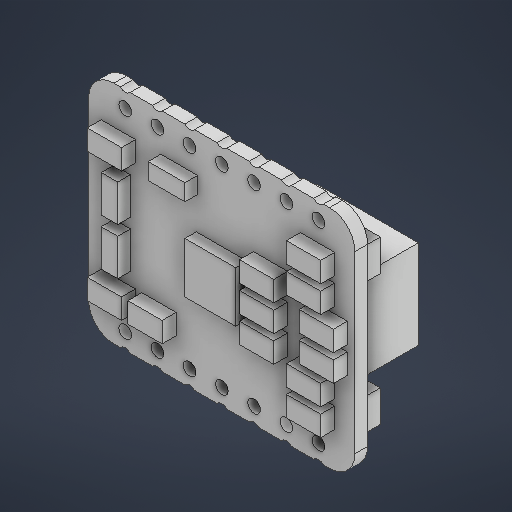
# Autodesk Inventor part: PCB
Saved by Autodesk Inventor 2027 (Build 310192000, 192)
## iProperties
Created: 2026-07-04
Part Number: PCB
Material: Genérico
Document SubType Name: Modeling
Designer: marcu
Density: 1 g/cm^3
Appearance: Padrão
Author: marcu
Autodesk Inventor part; units mm, degrees
ref_plane "YZ Plane" through (0, 0, 0) normal (1, 0, 0) x (0, 1, 0)
ref_plane "XZ Plane" through (0, 0, 0) normal (0, 1, 0) x (-1, 0, 0)
ref_plane "XY Plane" through (0, 0, 0) normal (0, 0, 1) x (1, 0, 0)
sketch "Esboço1" plane through (0, 0, 0) normal (0, 0, 1) x (1, 0, 0)
  line L0 (-10.5, 8.9) -> (10.5, 8.9)
  line L1 (10.5, 8.9) -> (10.5, -8.9)
  line L2 (10.5, -8.9) -> (-10.5, -8.9)
  line L3 (-10.5, -8.9) -> (-10.5, 8.9)
  line L4 (-10.5, 8.9) -> (10.5, -8.9) construction
  line L5 (10.5, 8.9) -> (-10.5, -8.9) construction
  point P0 (0, 0)
  dimension "d0" = 21
  dimension "d1" = 17.8
  constraints: 12 end point, 2 midpoint, 2 parallel, 1 horizontal, 1 perpendicular
  measures "d0" distance of L1.end L2.end
  measures "d1" distance of L0.end L1.end
extrude "Extrusão1" add sketch "Esboço1" along normal blind 1
fillet "Arredondamento1" radius 2 4 edges at (10.5, 8.9, 0.5) (10.5, -8.9, 0.5) (-10.5, -8.9, 0.5) (-10.5, 8.9, 0.5)
sketch "Esboço2" plane through (0, 0, 1) normal (0, 0, 1) x (1, 0, 0)
  line L0 (10.5, 8.9) -> (-10.5, 8.9) construction
  line L1 (-10.5, 8.9) -> (-10.5, -8.9) construction
  line L2 (-10.5, -8.9) -> (10.5, -8.9) construction
  line L3 (10.5, -8.9) -> (10.5, 8.9) construction
  line L4 (10.5, 8.9) -> (-10.5, -8.9) construction
  line L5 (-10.5, 8.9) -> (10.5, -8.9) construction
  circle A0 centre (7.63, -7.62) radius 0.5
  circle A1 centre (5.09, -7.62) radius 0.5
  circle A2 centre (2.55, -7.62) radius 0.5
  circle A3 centre (0.01, -7.62) radius 0.5
  circle A4 centre (-2.53, -7.62) radius 0.5
  circle A5 centre (-5.07, -7.62) radius 0.5
  circle A6 centre (-7.61, -7.62) radius 0.5
  line L6 (0, 0) -> (4.59, 0) construction
  circle A7 centre (7.63, 7.62) radius 0.5
  circle A8 centre (5.09, 7.62) radius 0.5
  circle A9 centre (2.55, 7.62) radius 0.5
  circle A10 centre (0.01, 7.62) radius 0.5
  circle A11 centre (-2.53, 7.62) radius 0.5
  circle A12 centre (-5.07, 7.62) radius 0.5
  circle A13 centre (-7.61, 7.62) radius 0.5
  dimension "d6" = 21
  dimension "d7" = 17.8
  dimension "d8" = 1
  dimension "d9" = 1.28
  dimension "d10" = 2.87
  dimension "d13" = 2.54
  constraints: 14 centre point, 14 end point, 7 symmetric about line, 3 horizontal, 2 midpoint, 2 parallel, 1 perpendicular, 19 other
  measures "d6" distance of L2.end L1.end
  measures "d7" distance of L1.end L0.end
  measures "d8" diameter of A0
  measures "d9" distance from line of L2 A0.centre
  measures "d10" distance from line of A0.centre L3
  measures "d13" distance of A0.centre A1.centre
extrude "Extrusão2" cut sketch "Esboço2" against normal blind 2
sketch "Esboço3" plane through (0, 0, 1) normal (0, 0, 1) x (1, 0, 0)
  circle A0 centre (7.63, -9.22) radius 0.5
  circle A1 centre (7.63, -7.62) radius 0.5 projected
  line L0 (8.6638, -8.12) -> (6.5962, -8.12) construction
  line L1 (8.6792, -8.72) -> (6.5808, -8.72) construction
  line L2 (-8.5, -8.9) -> (8.5, -8.9) projected
  line L3 (10.5, -6.9) -> (10.5, 6.9) projected
  circle A2 centre (5.09, -9.22) radius 0.5
  line L4 (6.1238, -8.12) -> (4.0562, -8.12) construction
  line L5 (6.1392, -8.72) -> (4.0408, -8.72) construction
  circle A3 centre (2.55, -9.22) radius 0.5
  line L6 (3.5838, -8.12) -> (1.5162, -8.12) construction
  line L7 (3.5992, -8.72) -> (1.5008, -8.72) construction
  circle A4 centre (0.01, -9.22) radius 0.5
  line L8 (1.0438, -8.12) -> (-1.0238, -8.12) construction
  line L9 (1.0592, -8.72) -> (-1.0392, -8.72) construction
  circle A5 centre (-2.53, -9.22) radius 0.5
  line L10 (-1.4962, -8.12) -> (-3.5638, -8.12) construction
  line L11 (-1.4808, -8.72) -> (-3.5792, -8.72) construction
  circle A6 centre (-5.07, -9.22) radius 0.5
  line L12 (-4.0362, -8.12) -> (-6.1038, -8.12) construction
  line L13 (-4.0208, -8.72) -> (-6.1192, -8.72) construction
  circle A7 centre (-7.61, -9.22) radius 0.5
  line L14 (-6.5762, -8.12) -> (-8.6438, -8.12) construction
  line L15 (-6.5608, -8.72) -> (-8.6592, -8.72) construction
  line L16 (2.53, 0) -> (-2.53, 0) construction
  circle A8 centre (7.63, 9.22) radius 0.5
  line L17 (8.6792, 8.72) -> (6.5808, 8.72) construction
  line L18 (-8.5, 8.9) -> (8.5, 8.9)
  circle A9 centre (5.09, 9.22) radius 0.5
  line L19 (6.1392, 8.72) -> (4.0408, 8.72) construction
  circle A10 centre (2.55, 9.22) radius 0.5
  line L20 (3.5992, 8.72) -> (1.5008, 8.72) construction
  circle A11 centre (0.01, 9.22) radius 0.5
  line L21 (1.0592, 8.72) -> (-1.0392, 8.72) construction
  circle A12 centre (-2.53, 9.22) radius 0.5
  line L22 (-1.4808, 8.72) -> (-3.5792, 8.72) construction
  circle A13 centre (-5.07, 9.22) radius 0.5
  line L23 (-4.0208, 8.72) -> (-6.1192, 8.72) construction
  circle A14 centre (-7.61, 9.22) radius 0.5
  line L24 (-6.5608, 8.72) -> (-8.6592, 8.72) construction
  point P0 (0, 0)
  point P1 (7.63, -8.12)
  point P2 (7.63, -8.72)
  point P3 (5.09, -8.72)
  point P4 (5.09, -8.12)
  point P5 (5.09, -7.62)
  point P6 (5.96, -8.9)
  point P7 (2.55, -8.72)
  point P8 (2.55, -8.12)
  point P9 (2.55, -7.62)
  point P10 (3.42, -8.9)
  point P11 (0.01, -8.72)
  point P12 (0.01, -8.12)
  point P13 (0.01, -7.62)
  point P14 (0.88, -8.9)
  point P15 (-2.53, -8.72)
  point P16 (-2.53, -8.12)
  point P17 (-2.53, -7.62)
  point P18 (-1.66, -8.9)
  point P19 (-5.07, -8.72)
  point P20 (-5.07, -8.12)
  point P21 (-5.07, -7.62)
  point P22 (-4.2, -8.9)
  point P23 (-7.61, -8.72)
  point P24 (-7.61, -8.12)
  point P25 (-7.61, -7.62)
  point P26 (-6.74, -8.9)
  point P27 (7.63, 8.72)
  point P28 (5.09, 8.72)
  point P29 (5.96, 8.9)
  point P30 (2.55, 8.72)
  point P31 (3.42, 8.9)
  point P32 (0.01, 8.72)
  point P33 (0.88, 8.9)
  point P34 (-2.53, 8.72)
  point P35 (-1.66, 8.9)
  point P36 (-5.07, 8.72)
  point P37 (-4.2, 8.9)
  point P38 (-7.61, 8.72)
  point P39 (-6.74, 8.9)
  dimension "d20" = 1
  dimension "d21" = 0.6
  dimension "d22" = 2.87
  dimension "d25" = 2.54
  constraints: 46 end point, 36 symmetric about line, 18 horizontal, 15 vertical alignment, 3 midpoint, 1 parallel, 95 other
  measures "d21" distance between parallel lines of L0 L1
  measures "d22" distance from line of point (7.63, -9.22) L3
  measures "d25" distance of point (7.63, -9.22) point (5.09, -9.22)
extrude "Extrusão3" cut sketch "Esboço3" against normal blind 2 contours A0 L2 | L2 A0 | A7 L2 | L2 A7 | A6 L2 | L2 A6 | A5 L2 | L2 A5 | A4 L2 | L2 A4 | A3 L2 | L2 A3 | A2 L2 | L2 A2 | A8 L18 | L18 A8 | A14 L18 | L18 A14 | A13 L18 | L18 A13 | A12 L18 | L18 A12 | A11 L18 | L18 A11 | A10 L18 | L18 A10 | A9 L18 | L18 A9
sketch "Esboço4" plane through (0, 0, 1) normal (0, 0, 1) x (1, 0, 0)
  line L0 (2, 2) -> (-2, 2)
  line L1 (-2, 2) -> (-2, -2)
  line L2 (-2, -2) -> (2, -2)
  line L3 (2, -2) -> (2, 2)
  line L4 (2, 2) -> (-2, -2) construction
  line L5 (-2, 2) -> (2, -2) construction
  point P0 (0, 0)
  dimension "d32" = 4
  dimension "d33" = 4
  constraints: 12 end point, 2 midpoint, 2 parallel, 1 horizontal, 1 perpendicular
  measures "d32" distance of L2.end L1.end
  measures "d33" distance of L1.end L0.end
extrude "MPU6050" add sketch "Esboço4" along normal blind 0.9
sketch "Esboço5" plane through (0, 0, 1) normal (0, 0, 1) x (1, 0, 0)
  line L0 (2, 2) -> (2, -2) projected
  line L1 (2.9342, -8.9) -> (4.7058, -8.9) projected
  line L2 (0, 2.9633) -> (0, -2.9633) construction
  line L3 (-2, 2) -> (-2, -2)
  line L4 (5.2, 2.9) -> (2.5, 2.9)
  line L5 (2.5, 2.9) -> (2.5, 1.3)
  line L6 (2.5, 1.3) -> (5.2, 1.3)
  line L7 (5.2, 1.3) -> (5.2, 2.9)
  line L8 (5.2, 2.9) -> (2.5, 1.3) construction
  line L9 (2.5, 2.9) -> (5.2, 1.3) construction
  line L10 (5.2, 0.8) -> (2.5, 0.8)
  line L11 (2.5, 0.8) -> (2.5, -0.8)
  line L12 (2.5, -0.8) -> (5.2, -0.8)
  line L13 (5.2, -0.8) -> (5.2, 0.8)
  line L14 (5.2, 0.8) -> (2.5, -0.8) construction
  line L15 (2.5, 0.8) -> (5.2, -0.8) construction
  line L16 (5.2, -1.3) -> (2.5, -1.3)
  line L17 (2.5, -1.3) -> (2.5, -2.9)
  line L18 (2.5, -2.9) -> (5.2, -2.9)
  line L19 (5.2, -2.9) -> (5.2, -1.3)
  line L20 (5.2, -1.3) -> (2.5, -2.9) construction
  line L21 (2.5, -1.3) -> (5.2, -2.9) construction
  point P0 (0, 0)
  point P1 (3.85, 2.1)
  point P2 (3.85, 0)
  point P3 (3.85, -2.1)
  dimension "d127" = 2.7
  dimension "d128" = 1.6
  dimension "d129" = 0.5
  dimension "d130" = 0.5
  dimension "d131" = 0.5
  dimension "d132" = 6
  constraints: 40 end point, 7 midpoint, 6 parallel, 4 equal length, 3 horizontal, 3 perpendicular, 2 point on line, 2 symmetric about line, 1 vertical
  measures "d127" distance of L6.end L5.end
  measures "d128" distance of L5.end L4.end
  measures "d129" distance between parallel lines of L6 L10
  measures "d130" distance between parallel lines of L12 L16
  measures "d131" distance between parallel lines of L0 L5
  measures "d132" distance between parallel lines of L1 L18
sketch "Esboço7" plane through (0, 0, 0) normal (0, 0, -1) x (-1, 0, 0)
  line L0 (-9, -3.5) -> (-1, -3.5)
  line L1 (-1, -3.5) -> (-1, 3.5)
  line L2 (-1, 3.5) -> (-9, 3.5)
  line L3 (-9, 3.5) -> (-9, -3.5)
  line L4 (-9, -3.5) -> (-1, 3.5) construction
  line L5 (-1, -3.5) -> (-9, 3.5) construction
  line L6 (-10.5, -6.9) -> (-10.5, 6.9) projected
  line L7 (-7.2458, 8.9) -> (-5.4742, 8.9) projected
  point P0 (0, 0)
  point P1 (-5, 0)
  dimension "d48" = 8
  dimension "d49" = 7
  dimension "d50" = 1.5
  dimension "d51" = 5.4
  constraints: 12 end point, 2 midpoint, 2 parallel, 1 horizontal, 1 perpendicular
  measures "d48" distance of L2.end L1.end
  measures "d49" distance of L1.end L0.end
  measures "d50" distance between parallel lines of L3 L6
  measures "d51" distance between parallel lines of L7 L2
extrude "JST" add sketch "Esboço7" along normal blind 5.5
sketch "Esboço8" plane through (0, 0, 0) normal (0, 0, -1) x (-1, 0, 0)
  line L0 (-10, 6.4) -> (-6.5, 6.4)
  line L1 (-6.5, 6.4) -> (-6.5, 3.9)
  line L2 (-6.5, 3.9) -> (-10, 3.9)
  line L3 (-10, 3.9) -> (-10, 6.4)
  line L4 (-10, 6.4) -> (-6.5, 3.9) construction
  line L5 (-6.5, 6.4) -> (-10, 3.9) construction
  line L6 (-10.5, -6.9) -> (-10.5, 6.9) projected
  line L7 (-8.5, 8.9) -> (-8.0142, 8.9) projected
  line L8 (-2, 0) -> (2, 0) construction
  line L9 (2, 2) -> (2, -2) projected
  line L10 (-10, -6.4) -> (-6.5, -6.4)
  line L11 (-6.5, -6.4) -> (-6.5, -3.9)
  line L12 (-6.5, -3.9) -> (-10, -3.9)
  line L13 (-10, -3.9) -> (-10, -6.4)
  line L14 (-10, -6.4) -> (-6.5, -3.9) construction
  line L15 (-6.5, -6.4) -> (-10, -3.9) construction
  line L16 (-8.5, -8.9) -> (-8.0142, -8.9)
  point P0 (0, 0)
  point P1 (-8.25, 5.15)
  point P2 (-8.25, -5.15)
  dimension "d54" = 3.5
  dimension "d55" = 2.5
  dimension "d56" = 0.5
  dimension "d57" = 2.5
  constraints: 28 end point, 7 symmetric about line, 4 midpoint, 2 parallel, 1 horizontal, 1 perpendicular
  measures "d54" distance of L1.end L2.end
  measures "d55" distance of L0.end L1.end
  measures "d56" distance between parallel lines of L6 L3
  measures "d57" distance between parallel lines of L0 L7
extrude "Botões Deslizantes" add sketch "Esboço8" along normal blind 1.5
sketch "Esboço9" plane through (0, 0, 0) normal (0, 0, -1) x (-1, 0, 0)
  line L0 (-0.5, -2.35) -> (1.5, -2.35)
  line L1 (1.5, -2.35) -> (1.5, -0.75)
  line L2 (1.5, -0.75) -> (-0.5, -0.75)
  line L3 (-0.5, -0.75) -> (-0.5, -2.35)
  line L4 (-0.5, -2.35) -> (1.5, -0.75) construction
  line L5 (1.5, -2.35) -> (-0.5, -0.75) construction
  line L6 (-0.5, 0.75) -> (1.5, 0.75)
  line L7 (1.5, 0.75) -> (1.5, 2.35)
  line L8 (1.5, 2.35) -> (-0.5, 2.35)
  line L9 (-0.5, 2.35) -> (-0.5, 0.75)
  line L10 (-0.5, 0.75) -> (1.5, 2.35) construction
  line L11 (1.5, 0.75) -> (-0.5, 2.35) construction
  line L12 (-1, 3.5) -> (-1, -3.5) projected
  line L13 (0.3742, 8.9) -> (2.1458, 8.9) projected
  line L14 (2, -1.7) -> (4, -1.7)
  line L15 (4, -1.7) -> (4, -0.1)
  line L16 (4, -0.1) -> (2, -0.1)
  line L17 (2, -0.1) -> (2, -1.7)
  line L18 (2, -1.7) -> (4, -0.1) construction
  line L19 (4, -1.7) -> (2, -0.1) construction
  line L20 (2, 0.1) -> (4, 0.1)
  line L21 (4, 0.1) -> (4, 1.7)
  line L22 (4, 1.7) -> (2, 1.7)
  line L23 (2, 1.7) -> (2, 0.1)
  line L24 (2, 0.1) -> (4, 1.7) construction
  line L25 (4, 0.1) -> (2, 1.7) construction
  line L26 (5.4542, 8.9) -> (7.2258, 8.9) projected
  point P0 (0, 0)
  point P1 (0.5, -1.55)
  point P2 (0.5, 1.55)
  point P3 (3, -0.9)
  point P4 (3, 0.9)
  dimension "d60" = 2
  dimension "d61" = 1.6
  dimension "d62" = 0.5
  dimension "d63" = 1.5
  dimension "d64" = 6.55
  dimension "d67" = 0.2
  dimension "d68" = 7.2
  dimension "d69" = 0.5
  dimension "d70" = 0.5
  constraints: 48 end point, 8 midpoint, 8 parallel, 6 equal length, 4 horizontal, 4 perpendicular, 1 point on line
  measures "d60" distance of L1.end L2.end
  measures "d61" distance of L0.start L2.end
  measures "d62" distance between parallel lines of L3 L12
  measures "d63" distance between parallel lines of L6 L2
  measures "d64" distance between parallel lines of L13 L8
  measures "d67" distance between parallel lines of L20 L16
  measures "d68" distance between parallel lines of L26 L22
  measures "d69" distance between parallel lines of L23 L7
  measures "d70" distance between parallel lines of L17 L1
extrude "capacitores" add sketch "Esboço9" along normal blind 1.6
sketch "Esboço10" plane through (0, 0, 0) normal (0, 0, -1) x (-1, 0, 0)
  line L0 (-0.8, -6.4) -> (0.8, -6.4)
  line L1 (0.8, -6.4) -> (0.8, -3.7)
  line L2 (0.8, -3.7) -> (-0.8, -3.7)
  line L3 (-0.8, -3.7) -> (-0.8, -6.4)
  line L4 (-0.8, -6.4) -> (0.8, -3.7) construction
  line L5 (0.8, -6.4) -> (-0.8, -3.7) construction
  line L6 (1.3, -6.4) -> (2.6, -6.4)
  line L7 (2.6, -6.4) -> (2.6, -3.5)
  line L8 (2.6, -3.5) -> (1.3, -3.5)
  line L9 (1.3, -3.5) -> (1.3, -6.4)
  line L10 (1.3, -6.4) -> (2.6, -3.5) construction
  line L11 (2.6, -6.4) -> (1.3, -3.5) construction
  line L12 (3.1, -6.4) -> (3.9, -6.4)
  line L13 (3.9, -6.4) -> (3.9, -4.8)
  line L14 (3.9, -4.8) -> (3.1, -4.8)
  line L15 (3.1, -4.8) -> (3.1, -6.4)
  line L16 (3.1, -6.4) -> (3.9, -4.8) construction
  line L17 (3.9, -6.4) -> (3.1, -4.8) construction
  line L18 (-1, 3.5) -> (-1, -3.5) projected
  line L19 (2.1458, -8.9) -> (0.3742, -8.9) projected
  line L20 (4.6858, -8.9) -> (2.9142, -8.9) projected
  line L21 (7.2258, -8.9) -> (5.4542, -8.9) projected
  line L22 (-1.26, 0) -> (1.26, 0) construction
  line L23 (-0.8, 6.4) -> (0.8, 6.4)
  line L24 (0.8, 6.4) -> (0.8, 3.7)
  line L25 (0.8, 3.7) -> (-0.8, 3.7)
  line L26 (-0.8, 3.7) -> (-0.8, 6.4)
  line L27 (-0.8, 6.4) -> (0.8, 3.7) construction
  line L28 (0.8, 6.4) -> (-0.8, 3.7) construction
  line L29 (1.3, 6.4) -> (2.6, 6.4)
  line L30 (2.6, 6.4) -> (2.6, 3.5)
  line L31 (2.6, 3.5) -> (1.3, 3.5)
  line L32 (1.3, 3.5) -> (1.3, 6.4)
  line L33 (1.3, 6.4) -> (2.6, 3.5) construction
  line L34 (2.6, 6.4) -> (1.3, 3.5) construction
  line L35 (3.1, 6.4) -> (3.9, 6.4)
  line L36 (3.9, 6.4) -> (3.9, 4.8)
  line L37 (3.9, 4.8) -> (3.1, 4.8)
  line L38 (3.1, 4.8) -> (3.1, 6.4)
  line L39 (3.1, 6.4) -> (3.9, 4.8) construction
  line L40 (3.9, 6.4) -> (3.1, 4.8) construction
  point P0 (0, 0)
  point P1 (0, -5.05)
  point P2 (1.95, -4.95)
  point P3 (3.5, -5.6)
  point P4 (0, 5.05)
  point P5 (1.95, 4.95)
  point P6 (3.5, 5.6)
  dimension "d73" = 1.6
  dimension "d74" = 2.7
  dimension "d75" = 1.3
  dimension "d76" = 2.9
  dimension "d77" = 0.8
  dimension "d78" = 1.6
  dimension "d79" = 0.2
  dimension "d80" = 2.5
  dimension "d81" = 2.5
  dimension "d82" = 2.5
  dimension "d83" = 0.5
  dimension "d84" = 0.5
  constraints: 74 end point, 15 symmetric about line, 7 midpoint, 6 parallel, 4 horizontal, 3 perpendicular
  measures "d73" distance of L2.end L1.end
  measures "d74" distance of L1.end L0.end
  measures "d75" distance of L8.end L7.end
  measures "d76" distance of L7.end L6.end
  measures "d77" distance of L14.end L13.end
  measures "d78" distance of L13.end L12.end
  measures "d79" distance between parallel lines of L3 L18
  measures "d80" distance between parallel lines of L19 L0
  measures "d81" distance between parallel lines of L20 L6
  measures "d82" distance between parallel lines of L21 L12
  measures "d83" distance between parallel lines of L9 L1
  measures "d84" distance between parallel lines of L15 L7
extrude "Diodo" add sketch "Esboço10" along normal blind 1.1 contours L3 L2 L1 L0 | L23 L24 L25 L26
extrude "Transistor" add sketch "Esboço10" along normal blind 1.1 contours L9 L8 L7 L6 | L29 L30 L31 L32
extrude "Resistor" add sketch "Esboço10" along normal blind 1.1 contours L15 L14 L13 L12 | L35 L36 L37 L38
sketch "Esboço11" plane through (0, 0, 0) normal (0, 0, -1) x (-1, 0, 0)
  line L0 (4.5, -3.7) -> (6.1, -3.7)
  line L1 (6.1, -3.7) -> (6.1, -1)
  line L2 (6.1, -1) -> (4.5, -1)
  line L3 (4.5, -1) -> (4.5, -3.7)
  line L4 (4.5, -3.7) -> (6.1, -1) construction
  line L5 (6.1, -3.7) -> (4.5, -1) construction
  line L6 (8.6, -2.6) -> (9.4, -2.6)
  line L7 (9.4, -2.6) -> (9.4, -1)
  line L8 (9.4, -1) -> (8.6, -1)
  line L9 (8.6, -1) -> (8.6, -2.6)
  line L10 (8.6, -2.6) -> (9.4, -1) construction
  line L11 (9.4, -2.6) -> (8.6, -1) construction
  line L12 (4, -0.1) -> (4, -1.7) projected
  line L13 (-1.0853, 0) -> (1.0853, 0) construction
  line L14 (6.7, -1) -> (8, -1)
  line L15 (8, -1) -> (8, -3.9)
  line L16 (8, -3.9) -> (6.7, -3.9)
  line L17 (6.7, -3.9) -> (6.7, -1)
  line L18 (6.7, -1) -> (8, -3.9) construction
  line L19 (8, -1) -> (6.7, -3.9) construction
  line L20 (4.5, 3.7) -> (6.1, 3.7)
  line L21 (6.1, 3.7) -> (6.1, 1)
  line L22 (6.1, 1) -> (4.5, 1)
  line L23 (4.5, 1) -> (4.5, 3.7)
  line L24 (4.5, 3.7) -> (6.1, 1) construction
  line L25 (6.1, 3.7) -> (4.5, 1) construction
  line L26 (8.6, 2.6) -> (9.4, 2.6)
  line L27 (9.4, 2.6) -> (9.4, 1)
  line L28 (9.4, 1) -> (8.6, 1)
  line L29 (8.6, 1) -> (8.6, 2.6)
  line L30 (8.6, 2.6) -> (9.4, 1) construction
  line L31 (9.4, 2.6) -> (8.6, 1) construction
  line L32 (6.7, 1) -> (8, 1)
  line L33 (8, 1) -> (8, 3.9)
  line L34 (8, 3.9) -> (6.7, 3.9)
  line L35 (6.7, 3.9) -> (6.7, 1)
  line L36 (6.7, 1) -> (8, 3.9) construction
  line L37 (8, 1) -> (6.7, 3.9) construction
  point P0 (0, 0)
  point P1 (5.3, -2.35)
  point P2 (9, -1.8)
  point P3 (7.35, -2.45)
  point P4 (5.3, 2.35)
  point P5 (9, 1.8)
  point P6 (4, 1.7)
  point P7 (7.35, 2.45)
  dimension "d101" = 2.7
  dimension "d102" = 1.6
  dimension "d105" = 1.6
  dimension "d106" = 0.8
  dimension "d107" = 1
  dimension "d108" = 1
  dimension "d109" = 1.3
  dimension "d110" = 2.9
  dimension "d111" = 1
  dimension "d112" = 0.6
  dimension "d113" = 0.6
  dimension "d114" = 0.5
  constraints: 74 end point, 16 symmetric about line, 7 midpoint, 6 parallel, 4 horizontal, 3 perpendicular
  measures "d101" distance of L2.end L0.start
  measures "d102" distance of L0.start L0.end
  measures "d105" distance of L8.end L6.start
  measures "d106" distance of L6.start L6.end
  measures "d107" distance from line of point (0, 0) L2
  measures "d108" distance from line of point (0, 0) L8
  measures "d109" distance of L15.end L16.end
  measures "d110" distance of L14.end L15.end
  measures "d111" distance from line of point (0, 0) L14
  measures "d112" distance between parallel lines of L17 L1
  measures "d113" distance between parallel lines of L9 L15
  measures "d114" distance between parallel lines of L12 L3
extrude "Extrusão12" add sketch "Esboço11" along normal blind 1.1 contours L3 L2 L1 L0 | L20 L21 L22 L23
extrude "Extrusão13" add sketch "Esboço11" along normal blind 1 contours L14 L15 L16 L17 | L35 L34 L33 L32
extrude "Extrusão14" add sketch "Esboço11" along normal blind 0.45 contours L9 L8 L7 L6 | L26 L27 L28 L29
sketch "Esboço12" plane through (0, 0, 0) normal (0, 0, -1) x (-1, 0, 0)
  line L0 (9.2, 5.8) -> (10, 5.8)
  line L1 (10, 5.8) -> (10, 7.4)
  line L2 (10, 7.4) -> (9.2, 7.4)
  line L3 (9.2, 7.4) -> (9.2, 5.8)
  line L4 (9.2, 5.8) -> (10, 7.4) construction
  line L5 (10, 5.8) -> (9.2, 7.4) construction
  line L6 (10.5, 6.9) -> (10.5, -6.9) projected
  line L7 (7.9942, 8.9) -> (8.5, 8.9) projected
  line L8 (-1.0954, 0) -> (1.0954, 0) construction
  line L9 (9.2, -5.8) -> (10, -5.8)
  line L10 (10, -5.8) -> (10, -7.4)
  line L11 (10, -7.4) -> (9.2, -7.4)
  line L12 (9.2, -7.4) -> (9.2, -5.8)
  line L13 (9.2, -5.8) -> (10, -7.4) construction
  line L14 (10, -5.8) -> (9.2, -7.4) construction
  point P0 (0, 0)
  point P1 (9.6, 6.6)
  point P2 (9.6, -6.6)
  dimension "d121" = 0.8
  dimension "d122" = 1.6
  dimension "d123" = 0.5
  dimension "d124" = 1.5
  constraints: 26 end point, 5 symmetric about line, 3 midpoint, 2 horizontal, 2 parallel, 1 perpendicular
  measures "d121" distance of L2.end L1.end
  measures "d122" distance of L1.end L0.end
  measures "d123" distance between parallel lines of L6 L1
  measures "d124" distance between parallel lines of L7 L2
extrude "LEDs" add sketch "Esboço12" along normal blind 0.6
extrude "Extrusão16" add sketch "Esboço5" along normal blind 1.1
sketch "Esboço13" plane through (0, 0, 1) normal (0, 0, 1) x (1, 0, 0)
  line L0 (8.9, 6.05) -> (6.2, 6.05)
  line L1 (6.2, 6.05) -> (6.2, 4.45)
  line L2 (6.2, 4.45) -> (8.9, 4.45)
  line L3 (8.9, 4.45) -> (8.9, 6.05)
  line L4 (8.9, 6.05) -> (6.2, 4.45) construction
  line L5 (6.2, 6.05) -> (8.9, 4.45) construction
  line L6 (8.9, 3.95) -> (6.2, 3.95)
  line L7 (6.2, 3.95) -> (6.2, 2.35)
  line L8 (6.2, 2.35) -> (8.9, 2.35)
  line L9 (8.9, 2.35) -> (8.9, 3.95)
  line L10 (8.9, 3.95) -> (6.2, 2.35) construction
  line L11 (6.2, 3.95) -> (8.9, 2.35) construction
  line L12 (9.9, 1.85) -> (7.2, 1.85)
  line L13 (7.2, 1.85) -> (7.2, 0.25)
  line L14 (7.2, 0.25) -> (9.9, 0.25)
  line L15 (9.9, 0.25) -> (9.9, 1.85)
  line L16 (9.9, 1.85) -> (7.2, 0.25) construction
  line L17 (7.2, 1.85) -> (9.9, 0.25) construction
  line L18 (9.9, -0.25) -> (7.2, -0.25)
  line L19 (7.2, -0.25) -> (7.2, -1.85)
  line L20 (7.2, -1.85) -> (9.9, -1.85)
  line L21 (9.9, -1.85) -> (9.9, -0.25)
  line L22 (9.9, -0.25) -> (7.2, -1.85) construction
  line L23 (7.2, -0.25) -> (9.9, -1.85) construction
  line L24 (8.9, -2.35) -> (6.2, -2.35)
  line L25 (6.2, -2.35) -> (6.2, -3.95)
  line L26 (6.2, -3.95) -> (8.9, -3.95)
  line L27 (8.9, -3.95) -> (8.9, -2.35)
  line L28 (8.9, -2.35) -> (6.2, -3.95) construction
  line L29 (6.2, -2.35) -> (8.9, -3.95) construction
  line L30 (8.9, -4.45) -> (6.2, -4.45)
  line L31 (6.2, -4.45) -> (6.2, -6.05)
  line L32 (6.2, -6.05) -> (8.9, -6.05)
  line L33 (8.9, -6.05) -> (8.9, -4.45)
  line L34 (8.9, -4.45) -> (6.2, -6.05) construction
  line L35 (6.2, -4.45) -> (8.9, -6.05) construction
  line L36 (5.2, 2.9) -> (5.2, 1.3) projected
  line L37 (5.2, -1.3) -> (5.2, -2.9) projected
  line L38 (7.2458, 8.9) -> (5.4742, 8.9) projected
  line L39 (5.2, 0.8) -> (5.2, -0.8) projected
  point P0 (0, 0)
  point P1 (7.55, 5.25)
  point P2 (7.55, 3.15)
  point P3 (8.55, 1.05)
  point P4 (8.55, -1.05)
  point P5 (7.55, -3.15)
  point P6 (7.55, -5.25)
  dimension "d135" = 2.7
  dimension "d136" = 1.6
  dimension "d137" = 2.7
  dimension "d138" = 1.6
  dimension "d139" = 2.7
  dimension "d140" = 1.6
  dimension "d141" = 2.7
  dimension "d142" = 1.6
  dimension "d143" = 2.7
  dimension "d144" = 1.6
  dimension "d145" = 2.7
  dimension "d146" = 1.6
  dimension "d147" = 1
  dimension "d148" = 1
  dimension "d149" = 1
  dimension "d150" = 1
  dimension "d151" = 2.85
  dimension "d152" = 0.5
  dimension "d153" = 0.5
  dimension "d154" = 0.5
  dimension "d155" = 0.5
  dimension "d156" = 0.5
  dimension "d157" = 2
  dimension "d158" = 2
  constraints: 72 end point, 12 midpoint, 12 parallel, 6 horizontal, 6 perpendicular
  measures "d135" distance of L2.end L1.end
  measures "d136" distance of L1.end L0.end
  measures "d137" distance of L8.end L7.end
  measures "d138" distance of L7.end L6.end
  measures "d139" distance of L14.end L13.end
  measures "d140" distance of L13.end L12.end
  measures "d141" distance of L20.end L19.end
  measures "d142" distance of L19.end L18.end
  measures "d143" distance of L26.end L25.end
  measures "d144" distance of L25.end L24.end
  measures "d145" distance of L32.end L31.end
  measures "d146" distance of L31.end L30.end
  measures "d147" distance between parallel lines of L36 L1
  measures "d148" distance between parallel lines of L36 L7
  measures "d149" distance between parallel lines of L37 L25
  measures "d150" distance between parallel lines of L37 L31
  measures "d151" distance between parallel lines of L38 L0
  measures "d152" distance between parallel lines of L2 L6
  measures "d153" distance between parallel lines of L8 L12
  measures "d154" distance between parallel lines of L14 L18
  measures "d155" distance between parallel lines of L20 L24
  measures "d156" distance between parallel lines of L26 L30
  measures "d157" distance between parallel lines of L39 L19
  measures "d158" distance between parallel lines of L36 L13
extrude "Extrusão17" add sketch "Esboço13" along normal blind 1.1
sketch "Esboço14" plane through (0, 0, 1) normal (0, 0, 1) x (1, 0, 0)
  line L0 (-3.6, -4.3) -> (-6.3, -4.3)
  line L1 (-6.3, -4.3) -> (-6.3, -5.9)
  line L2 (-6.3, -5.9) -> (-3.6, -5.9)
  line L3 (-3.6, -5.9) -> (-3.6, -4.3)
  line L4 (-3.6, -4.3) -> (-6.3, -5.9) construction
  line L5 (-6.3, -4.3) -> (-3.6, -5.9) construction
  line L6 (-6.8, -4.3) -> (-9.5, -4.3)
  line L7 (-9.5, -4.3) -> (-9.5, -5.9)
  line L8 (-9.5, -5.9) -> (-6.8, -5.9)
  line L9 (-6.8, -5.9) -> (-6.8, -4.3)
  line L10 (-6.8, -4.3) -> (-9.5, -5.9) construction
  line L11 (-9.5, -4.3) -> (-6.8, -5.9) construction
  line L12 (-10.5, 6.9) -> (-10.5, -6.9) projected
  line L13 (-4.6858, -8.9) -> (-2.9142, -8.9) projected
  line L14 (-8.5, -8.9) -> (-7.9942, -8.9) projected
  line L15 (-7.2, -0.4) -> (-8.5, -0.4)
  line L16 (-8.5, -0.4) -> (-8.5, -3.3)
  line L17 (-8.5, -3.3) -> (-7.2, -3.3)
  line L18 (-7.2, -3.3) -> (-7.2, -0.4)
  line L19 (-7.2, -0.4) -> (-8.5, -3.3) construction
  line L20 (-8.5, -0.4) -> (-7.2, -3.3) construction
  line L21 (4.6858, 0) -> (-4.6858, 0) construction
  line L22 (-6.8, 4.3) -> (-9.5, 4.3)
  line L23 (-9.5, 4.3) -> (-9.5, 5.9)
  line L24 (-9.5, 5.9) -> (-6.8, 5.9)
  line L25 (-6.8, 5.9) -> (-6.8, 4.3)
  line L26 (-6.8, 4.3) -> (-9.5, 5.9) construction
  line L27 (-9.5, 4.3) -> (-6.8, 5.9) construction
  line L28 (-7.2, 0.4) -> (-8.5, 0.4)
  line L29 (-8.5, 0.4) -> (-8.5, 3.3)
  line L30 (-8.5, 3.3) -> (-7.2, 3.3)
  line L31 (-7.2, 3.3) -> (-7.2, 0.4)
  line L32 (-7.2, 0.4) -> (-8.5, 3.3) construction
  line L33 (-8.5, 0.4) -> (-7.2, 3.3) construction
  line L34 (-1.9, 5.9) -> (-4.8, 5.9)
  line L35 (-4.8, 5.9) -> (-4.8, 4.6)
  line L36 (-4.8, 4.6) -> (-1.9, 4.6)
  line L37 (-1.9, 4.6) -> (-1.9, 5.9)
  line L38 (-1.9, 5.9) -> (-4.8, 4.6) construction
  line L39 (-4.8, 5.9) -> (-1.9, 4.6) construction
  line L40 (-2.9142, 8.9) -> (-4.6858, 8.9) projected
  point P0 (0, 0)
  point P1 (-4.95, -5.1)
  point P2 (-8.15, -5.1)
  point P3 (-7.85, -1.85)
  point P4 (-8.15, 5.1)
  point P5 (-7.85, 1.85)
  point P6 (-3.35, 5.25)
  dimension "d161" = 2.7
  dimension "d162" = 1.6
  dimension "d163" = 2.7
  dimension "d164" = 1.6
  dimension "d165" = 0.5
  dimension "d166" = 1
  dimension "d167" = 3
  dimension "d168" = 3
  dimension "d169" = 1.3
  dimension "d170" = 2.9
  dimension "d171" = 1
  dimension "d172" = 2
  dimension "d173" = 2.9
  dimension "d174" = 1.3
  dimension "d175" = 3
  dimension "d176" = 2
  constraints: 74 end point, 10 symmetric about line, 9 midpoint, 8 parallel, 5 horizontal, 4 perpendicular
  measures "d161" distance of L2.end L1.end
  measures "d162" distance of L1.end L0.end
  measures "d163" distance of L8.end L7.end
  measures "d164" distance of L7.end L6.end
  measures "d165" distance between parallel lines of L9 L1
  measures "d166" distance between parallel lines of L12 L7
  measures "d167" distance between parallel lines of L13 L2
  measures "d168" distance between parallel lines of L14 L8
  measures "d169" distance of L17.end L16.end
  measures "d170" distance of L16.end L15.end
  measures "d171" distance between parallel lines of L0 L17
  measures "d172" distance between parallel lines of L12 L16
  measures "d173" distance of L36.end L35.end
  measures "d174" distance of L35.end L34.end
  measures "d175" distance between parallel lines of L40 L34
  measures "d176" distance between parallel lines of L25 L35
extrude "Extrusão18" add sketch "Esboço14" along normal blind 1.1 contours L3 L2 L1 L0 | L9 L8 L7 L6 | L22 L23 L24 L25
extrude "Extrusão19" add sketch "Esboço14" along normal blind 1 contours L18 L17 L16 L15 | L28 L29 L30 L31 | L37 L36 L35 L34
